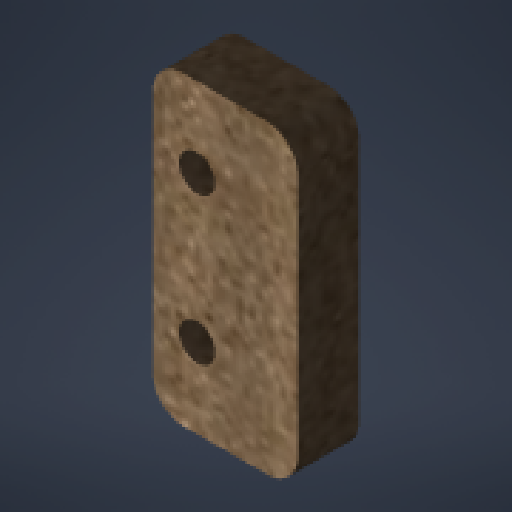
# Autodesk Inventor part: Door_LimitSwitch_Offset
Saved by Autodesk Inventor 2024.1 (Build 281209000, 209)
## iProperties
Created: 2023-08-05
Part Number: Door_LimitSwitch_Offset
Material: MDF Medium Density Fiberboard
Document SubType Name: Modeling
Designer: jaege
Density: 0.8 g/cm^3
Appearance: Cardboard - Corrugated
Author: jaege
Autodesk Inventor part; units mm, degrees
ref_plane "YZ Plane" through (0, 0, 0) normal (1, 0, 0) x (0, 1, 0)
ref_plane "XZ Plane" through (0, 0, 0) normal (0, 1, 0) x (-1, 0, 0)
ref_plane "XY Plane" through (0, 0, 0) normal (0, 0, 1) x (1, 0, 0)
sketch "Sketch1" plane through (0, 0, 0) normal (0, 0, 1) x (1, 0, 0)
  line L0 (-17.9772, -42.3695) -> (-21.9772, -42.3695) construction
  line L1 (-21.9772, -42.3695) -> (-21.9772, -36.3695) construction
  line L2 (-21.9772, -36.3695) -> (-17.9772, -36.3695) construction
  line L3 (-17.9772, -36.3695) -> (-17.9772, -42.3695) construction
  line L4 (52, -0.656) -> (44, -0.656) construction
  line L5 (44, -0.656) -> (44, 3.344) construction
  line L6 (44, 3.344) -> (52, 3.344) construction
  line L7 (52, 3.344) -> (52, -0.656) construction
  line L8 (-62, 48.621) -> (-62, 52.621) construction
  line L9 (-62, 52.621) -> (-54, 52.621) construction
  line L10 (-54, 52.621) -> (-54, 48.621) construction
  line L11 (-54, 48.621) -> (-62, 48.621) construction
  line L12 (-52, 7.344) -> (-52, 11.344) construction
  line L13 (-52, 11.344) -> (-44, 11.344) construction
  line L14 (-44, 11.344) -> (-44, 7.344) construction
  line L15 (-44, 7.344) -> (-52, 7.344) construction
  line L16 (62, 52.621) -> (62, 48.621) construction
  line L17 (62, 48.621) -> (54, 48.621) construction
  line L18 (54, 48.621) -> (54, 52.621) construction
  line L19 (54, 52.621) -> (62, 52.621) construction
  line L20 (44, 7.344) -> (44, 11.344) construction
  line L21 (44, 11.344) -> (52, 11.344) construction
  line L22 (52, 11.344) -> (52, 7.344) construction
  line L23 (52, 7.344) -> (44, 7.344) construction
  line L24 (-62, 56.621) -> (-62, 60.621) construction
  line L25 (-62, 60.621) -> (-54, 60.621) construction
  line L26 (-54, 60.621) -> (-54, 56.621) construction
  line L27 (-54, 56.621) -> (-62, 56.621) construction
  line L28 (-52, -0.656) -> (-52, 3.344) construction
  line L29 (-52, 3.344) -> (-44, 3.344) construction
  line L30 (-44, 3.344) -> (-44, -0.656) construction
  line L31 (-44, -0.656) -> (-52, -0.656) construction
  line L32 (62, 56.621) -> (54, 56.621) construction
  line L33 (54, 56.621) -> (54, 60.621) construction
  line L34 (54, 60.621) -> (62, 60.621) construction
  line L35 (62, 60.621) -> (62, 56.621) construction
  line L36 (95, 92.776) -> (95, 67.276) construction
  line L37 (-95, 92.776) -> (95, 92.776) construction
  line L38 (-95, 67.276) -> (-95, 92.776) construction
  spline S0 degree 4 poles (-93.2021, 32.276) (-94.3974, 41.3088) (-94.1998, 50.4639) (-95, 58.5765) (-95, 67.276) knots 0 0 0 0 0 1 1 1 1 1 construction
  spline S1 degree 3 poles (-93.2021, 32.276) (-92.477, 26.7964) (-92.3858, 18.3442) (-91.1679, 2.9086) (-90.2735, -4.0991) (-87.5297, -12.5723) (-86.3245, -15.3658) (-83.5784, -19.0417) (-82.333, -20.2665) (-79.6267, -21.887) (-78.3236, -22.3544) (-75.4283, -22.8138) (-73.9041, -22.7525) (-70.1581, -22.0875) (-67.9924, -21.2389) (-63.108, -18.9118) (-60.4378, -17.2966) (-54.8519, -14.6799) (-51.0186, -13.1408) (-44.4768, -12.6137) (-42.1843, -12.7653) (-38.5465, -13.8837) (-37.172, -14.5679) (-34.6876, -16.441) (-33.6448, -17.5823) (-32.7756, -18.8783) knots 0 0 0 0 1.658209 1.658209 2.939775 2.939775 3.538541 3.538541 3.905679 3.905679 4.202372 4.202372 4.52291 4.52291 5.00118 5.00118 5.654804 5.654804 6.203864 6.203864 6.490865 6.490865 6.688319 6.688319 6.886783 6.886783 6.886783 6.886783 construction
  spline S2 degree 4 poles (95, 67.276) (95, 55.7504) (92.5859, 37.7114) (100.8312, 0.406) (16.3507, -5.0368) (37.7982, -57.0134) (0, -92.776) (-31.6805, -62.8016) (-26.5791, -34.2881) (-31.0379, -21.8211) (-32.7756, -18.8783) knots 0 0 0 0 0 0.141322 0.242902 0.345989 0.449799 0.550201 0.654011 0.69056 0.69056 0.69056 0.69056 0.69056 construction
  line L39 (-40, 82.776) -> (-44, 82.776) construction
  line L40 (-40, 62.776) -> (-40, 82.776) construction
  line L41 (-44, 62.776) -> (-40, 62.776) construction
  line L42 (-44, 82.776) -> (-44, 62.776) construction
  line L43 (-40, 22.776) -> (-40, 42.776) construction
  line L44 (-44, 22.776) -> (-40, 22.776) construction
  line L45 (-44, 42.776) -> (-44, 22.776) construction
  line L46 (-40, 42.776) -> (-44, 42.776) construction
  line L47 (-10, 12.776) -> (-30, 12.776) construction
  line L48 (-10, 8.776) -> (-10, 12.776) construction
  line L49 (-30, 8.776) -> (-10, 8.776) construction
  line L50 (-30, 12.776) -> (-30, 8.776) construction
  line L51 (44, 82.776) -> (40, 82.776) construction
  line L52 (44, 62.776) -> (44, 82.776) construction
  line L53 (40, 62.776) -> (44, 62.776) construction
  line L54 (40, 82.776) -> (40, 62.776) construction
  line L55 (44, 22.776) -> (44, 42.776) construction
  line L56 (40, 22.776) -> (44, 22.776) construction
  line L57 (40, 42.776) -> (40, 22.776) construction
  line L58 (44, 42.776) -> (40, 42.776) construction
  line L59 (30, 12.776) -> (10, 12.776) construction
  line L60 (30, 8.776) -> (30, 12.776) construction
  line L61 (10, 8.776) -> (30, 8.776) construction
  line L62 (10, 12.776) -> (10, 8.776) construction
  circle A0 centre (-78.75, 27.8364) radius 1.5 construction
  circle A1 centre (-58.125, 15.9285) radius 1.5 construction
  circle A2 centre (-71.875, 15.9285) radius 1.5 construction
  circle A3 centre (-71.875, 39.7442) radius 1.5 construction
  circle A4 centre (-58.125, 39.7442) radius 1.5 construction
  circle A5 centre (-51.25, 27.8364) radius 1.5 construction
  circle A6 centre (-65, 27.8364) radius 10.5 construction
  circle A7 centre (-8.625, -30.663) radius 1.5 construction
  circle A8 centre (8.625, -30.663) radius 1.5 construction
  circle A9 centre (17.25, -15.724) radius 1.5 construction
  circle A10 centre (8.625, -0.7851) radius 1.5 construction
  circle A11 centre (-8.625, -0.7851) radius 1.5 construction
  circle A12 centre (-17.25, -15.724) radius 1.5 construction
  circle A13 centre (6.875, -45.3162) radius 1.5 construction
  circle A14 centre (13.75, -57.224) radius 1.5 construction
  circle A15 centre (0, -57.224) radius 10.5 construction
  circle A16 centre (-6.875, -69.1319) radius 1.5 construction
  circle A17 centre (6.875, -69.1319) radius 1.5 construction
  circle A18 centre (-6.875, -45.3162) radius 1.5 construction
  circle A19 centre (-13.75, -57.224) radius 1.5 construction
  circle A20 centre (58.125, 15.9285) radius 1.5 construction
  circle A21 centre (71.875, 15.9285) radius 1.5 construction
  circle A22 centre (78.75, 27.8364) radius 1.5 construction
  circle A23 centre (71.875, 39.7442) radius 1.5 construction
  circle A24 centre (58.125, 39.7442) radius 1.5 construction
  circle A25 centre (51.25, 27.8364) radius 1.5 construction
  circle A26 centre (0, -15.724) radius 14 construction
  circle A27 centre (65, 27.8364) radius 10.5 construction
  circle A28 centre (8.9, 77.626) radius 1.175
  circle A29 centre (8.9, 68.126) radius 1.175
  line L63 (6, 62.976) -> (15.4, 62.976)
  line L64 (15.4, 62.976) -> (15.4, 82.776)
  line L65 (15.4, 82.776) -> (6, 82.776)
  line L66 (6, 82.776) -> (6, 62.976)
  point P0 (0, 0)
  dimension "d0" = 24.6
  dimension "d1" = 2.35
  dimension "d2" = 9.5
  dimension "d3" = 19.8
  dimension "d4" = 9.4
  dimension "d5" = 5.15
  dimension "d6" = 2.9
  dimension "d7" = 10
  constraints: 8 end point, 2 centre point, 2 parallel, 1 equal radius, 1 horizontal, 1 perpendicular, 1 vertical alignment
  measures "d0" distance between parallel lines of L54 L64
  measures "d1" diameter of A28
  measures "d2" distance of A29.centre A28.centre
  measures "d3" distance of L63.end L64.end
  measures "d4" distance of L64.end L65.end
  measures "d5" distance from line of L65 A28.centre
  measures "d6" distance from line of L66 A28.centre
  measures "d7" distance between parallel lines of L37 L65
extrude "Extrusion1" add sketch "Sketch1" along normal blind 4
fillet "Fillet1" radius 2 4 edges at (6, 62.976, 2) (15.4, 62.976, 2) (15.4, 82.776, 2) (6, 82.776, 2)
body "Solid1"
